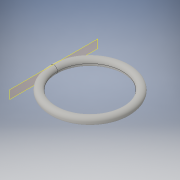
# Autodesk Inventor part: mcdave_oring
Saved by Autodesk Inventor 2016 (Build 200138000, 138)
## iProperties
Created: 2017-09-12
Part Number: mcdave_oring
Material: Generic
Document SubType Name: Modeling
Designer: student
Density: 1 g/cm^3
Appearance: Default
Author: student
Autodesk Inventor part; units mm, degrees
ref_plane "XZ Plane" through (0, 0, 0) normal (0, 1, 0) x (-1, 0, 0)
ref_plane "XY Plane" through (0, 0, 0) normal (0, 0, 1) x (1, 0, 0)
sketch "Sketch1" plane through (0, 0, 0) normal (0, 0, 1) x (1, 0, 0)
  circle A0 centre (0, 0) radius 2.5019
  dimension "d0" = 5.0038
  constraints: 1 centre point, 1 coincident
  measures "d0" diameter of A0
sketch "Sketch2" plane through (0, 0, 0) normal (0, 1, 0) x (-1, 0, 0)
  circle A0 centre (-23.6296, -0.8715) radius 23.5712
  point P0 (0, 0)
  dimension "d1" = 47.1424
  constraints: 1 centre point
  measures "d1" diameter of A0
sweep "Sweep1" add profiles "Sketch1" path "Sketch2"
body "Solid1"
